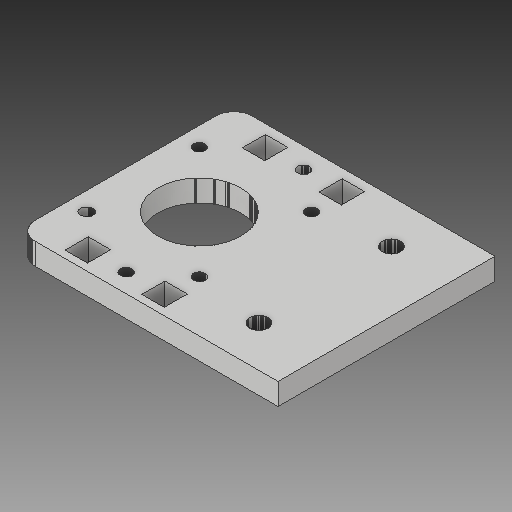
# Autodesk Inventor part: Y-Motor-Mount Top
Saved by Autodesk Inventor 2018 (Build 220112000, 112)
## iProperties
Created: 2016-07-22
Part Number: Y-Motor-Mount Top
Material: Generic
Document SubType Name: Modeling
Designer: User
Density: 1 g/cm^3
Appearance: Default
Mass: 21.9439 g
Surface Area: 104.712 cm^2
Volume: 21.9439 cm^3
Author: User
Autodesk Inventor part; units mm, degrees
ref_plane "YZ Plane" through (0, 0, 0) normal (1, 0, 0) x (0, 1, 0)
ref_plane "XZ Plane" through (0, 0, 0) normal (0, 1, 0) x (-1, 0, 0)
ref_plane "XY Plane" through (0, 0, 0) normal (0, 0, 1) x (1, 0, 0)
sketch "Sketch1" plane through (0, 0, 0) normal (0, 1, 0) x (-1, 0, 0)
  line L0 (968.8679, 195.3235) -> (968.6178, 195.9235)
  line L1 (968.6178, 195.9235) -> (968.2179, 196.4485)
  line L2 (968.2179, 196.4485) -> (967.6929, 196.8485)
  line L3 (967.6929, 196.8485) -> (967.0929, 197.0985)
  line L4 (967.0929, 197.0985) -> (966.4429, 197.1985)
  line L5 (966.4429, 197.1985) -> (965.7929, 197.0984)
  line L6 (965.7929, 197.0984) -> (965.1679, 196.8484)
  line L7 (965.1679, 196.8484) -> (964.6429, 196.4484)
  line L8 (964.6429, 196.4484) -> (964.2429, 195.9234)
  line L9 (964.2429, 195.9234) -> (963.9929, 195.3234)
  line L10 (963.9929, 195.3234) -> (963.9179, 194.6734)
  line L11 (963.9179, 194.6734) -> (963.9929, 194.0234)
  line L12 (963.9929, 194.0234) -> (964.243, 193.3984)
  line L13 (964.243, 193.3984) -> (964.6429, 192.8984)
  line L14 (964.6429, 192.8984) -> (965.1679, 192.4985)
  line L15 (965.1679, 192.4985) -> (965.793, 192.2485)
  line L16 (965.793, 192.2485) -> (966.443, 192.1486)
  line L17 (966.443, 192.1486) -> (967.093, 192.2486)
  line L18 (967.093, 192.2486) -> (967.6929, 192.4987)
  line L19 (967.6929, 192.4987) -> (968.218, 192.8987)
  line L20 (968.218, 192.8987) -> (968.6181, 193.3986)
  line L21 (968.6181, 193.3986) -> (968.868, 194.0236)
  line L22 (968.868, 194.0236) -> (968.9429, 194.6733)
  line L23 (968.9429, 194.6733) -> (968.8679, 195.3235)
  line L24 (983.267, 191.6734) -> (983.267, 185.2734)
  line L25 (983.267, 185.2734) -> (989.467, 185.2734)
  line L26 (989.467, 185.2734) -> (989.467, 191.6734)
  line L27 (989.467, 191.6734) -> (983.267, 191.6734)
  line L28 (987.3418, 197.698) -> (987.3418, 197.798)
  line L29 (987.3418, 197.798) -> (987.3169, 197.898)
  line L30 (987.3169, 197.898) -> (987.2669, 197.998)
  line L31 (987.2669, 197.998) -> (987.2419, 198.098)
  line L32 (987.2419, 198.098) -> (987.1919, 198.198)
  line L33 (987.1919, 198.198) -> (987.1419, 198.298)
  line L34 (987.1419, 198.298) -> (987.0919, 198.373)
  line L35 (987.0919, 198.373) -> (987.042, 198.473)
  line L36 (987.042, 198.473) -> (986.9669, 198.548)
  line L37 (986.9669, 198.548) -> (986.892, 198.6231)
  line L38 (986.892, 198.6231) -> (986.817, 198.6981)
  line L39 (986.817, 198.6981) -> (986.742, 198.7481)
  line L40 (986.742, 198.7481) -> (986.642, 198.8231)
  line L41 (986.642, 198.8231) -> (986.567, 198.8731)
  line L42 (986.567, 198.8731) -> (986.467, 198.9232)
  line L43 (986.467, 198.9232) -> (986.3671, 198.9732)
  line L44 (986.3671, 198.9732) -> (986.2671, 198.9983)
  line L45 (986.2671, 198.9983) -> (986.1671, 199.0483)
  line L46 (986.1671, 199.0483) -> (986.0671, 199.0483)
  line L47 (986.0671, 199.0483) -> (985.9671, 199.0734)
  line L48 (985.9671, 199.0734) -> (985.8671, 199.0983)
  line L49 (985.8671, 199.0983) -> (985.7671, 199.0983)
  line L50 (985.7671, 199.0983) -> (985.6671, 199.0983)
  line L51 (985.6671, 199.0983) -> (985.5422, 199.0734)
  line L52 (985.5422, 199.0734) -> (985.4421, 199.0483)
  line L53 (985.4421, 199.0483) -> (985.3421, 199.0483)
  line L54 (985.3421, 199.0483) -> (985.2421, 198.9983)
  line L55 (985.2421, 198.9983) -> (985.1421, 198.9733)
  line L56 (985.1421, 198.9733) -> (985.0421, 198.9234)
  line L57 (985.0421, 198.9234) -> (984.9671, 198.8733)
  line L58 (984.9671, 198.8733) -> (984.8671, 198.8234)
  line L59 (984.8671, 198.8234) -> (984.7922, 198.7484)
  line L60 (984.7922, 198.7484) -> (984.7171, 198.6984)
  line L61 (984.7171, 198.6984) -> (984.6421, 198.6234)
  line L62 (984.6421, 198.6234) -> (984.5671, 198.5484)
  line L63 (984.5671, 198.5484) -> (984.4921, 198.4734)
  line L64 (984.4921, 198.4734) -> (984.4421, 198.3734)
  line L65 (984.4421, 198.3734) -> (984.3671, 198.2984)
  line L66 (984.3671, 198.2984) -> (984.317, 198.1984)
  line L67 (984.317, 198.1984) -> (984.292, 198.0984)
  line L68 (984.292, 198.0984) -> (984.2421, 197.9984)
  line L69 (984.2421, 197.9984) -> (984.2171, 197.8985)
  line L70 (984.2171, 197.8985) -> (984.192, 197.7984)
  line L71 (984.192, 197.7984) -> (984.167, 197.6984)
  line L72 (984.167, 197.6984) -> (984.167, 197.5984)
  line L73 (984.167, 197.5984) -> (984.167, 197.4984)
  line L74 (984.167, 197.4984) -> (984.167, 197.3984)
  line L75 (984.167, 197.3984) -> (984.167, 197.2734)
  line L76 (984.167, 197.2734) -> (984.192, 197.1734)
  line L77 (984.192, 197.1734) -> (984.2171, 197.0734)
  line L78 (984.2171, 197.0734) -> (984.2421, 196.9734)
  line L79 (984.2421, 196.9734) -> (984.2921, 196.8734)
  line L80 (984.2921, 196.8734) -> (984.317, 196.7734)
  line L81 (984.317, 196.7734) -> (984.3671, 196.6985)
  line L82 (984.3671, 196.6985) -> (984.4421, 196.5985)
  line L83 (984.4421, 196.5985) -> (984.4921, 196.5235)
  line L84 (984.4921, 196.5235) -> (984.5671, 196.4235)
  line L85 (984.5671, 196.4235) -> (984.6421, 196.3485)
  line L86 (984.6421, 196.3485) -> (984.7171, 196.2984)
  line L87 (984.7171, 196.2984) -> (984.7921, 196.2234)
  line L88 (984.7921, 196.2234) -> (984.867, 196.1484)
  line L89 (984.867, 196.1484) -> (984.967, 196.0983)
  line L90 (984.967, 196.0983) -> (985.042, 196.0483)
  line L91 (985.042, 196.0483) -> (985.142, 196.0233)
  line L92 (985.142, 196.0233) -> (985.2419, 195.9732)
  line L93 (985.2419, 195.9732) -> (985.3419, 195.9482)
  line L94 (985.3419, 195.9482) -> (985.4419, 195.9231)
  line L95 (985.4419, 195.9231) -> (985.542, 195.8981)
  line L96 (985.542, 195.8981) -> (985.6669, 195.8981)
  line L97 (985.6669, 195.8981) -> (985.7669, 195.8981)
  line L98 (985.7669, 195.8981) -> (985.8669, 195.8981)
  line L99 (985.8669, 195.8981) -> (985.9669, 195.8981)
  line L100 (985.9669, 195.8981) -> (986.0669, 195.9231)
  line L101 (986.0669, 195.9231) -> (986.1669, 195.9481)
  line L102 (986.1669, 195.9481) -> (986.2669, 195.9731)
  line L103 (986.2669, 195.9731) -> (986.3669, 196.0231)
  line L104 (986.3669, 196.0231) -> (986.4669, 196.0482)
  line L105 (986.4669, 196.0482) -> (986.5669, 196.0981)
  line L106 (986.5669, 196.0981) -> (986.6419, 196.1481)
  line L107 (986.6419, 196.1481) -> (986.7419, 196.2231)
  line L108 (986.7419, 196.2231) -> (986.8169, 196.2981)
  line L109 (986.8169, 196.2981) -> (986.8919, 196.3481)
  line L110 (986.8919, 196.3481) -> (986.9669, 196.4231)
  line L111 (986.9669, 196.4231) -> (987.042, 196.5231)
  line L112 (987.042, 196.5231) -> (987.092, 196.5981)
  line L113 (987.092, 196.5981) -> (987.1419, 196.6981)
  line L114 (987.1419, 196.6981) -> (987.192, 196.7731)
  line L115 (987.192, 196.7731) -> (987.242, 196.8731)
  line L116 (987.242, 196.8731) -> (987.267, 196.9731)
  line L117 (987.267, 196.9731) -> (987.3169, 197.0731)
  line L118 (987.3169, 197.0731) -> (987.3419, 197.1731)
  line L119 (987.3419, 197.1731) -> (987.3419, 197.2731)
  line L120 (987.3419, 197.2731) -> (987.3669, 197.398)
  line L121 (987.3669, 197.398) -> (987.3669, 197.4979)
  line L122 (987.3669, 197.4979) -> (987.3669, 197.598)
  line L123 (987.3669, 197.598) -> (987.3418, 197.698)
  line L124 (1012.7431, 213.7485) -> (1012.6681, 214.4985)
  line L125 (1012.6681, 214.4985) -> (1012.5425, 215.2239)
  line L126 (1012.5425, 215.2239) -> (1012.3674, 215.9738)
  line L127 (1012.3674, 215.9738) -> (1012.1423, 216.6988)
  line L128 (1012.1423, 216.6988) -> (1011.8923, 217.3988)
  line L129 (1011.8923, 217.3988) -> (1011.5673, 218.0738)
  line L130 (1011.5673, 218.0738) -> (1011.2173, 218.7488)
  line L131 (1011.2173, 218.7488) -> (1010.8173, 219.3738)
  line L132 (1010.8173, 219.3738) -> (1010.3922, 219.9987)
  line L133 (1010.3922, 219.9987) -> (1009.917, 220.5735)
  line L134 (1009.917, 220.5735) -> (1009.3919, 221.1234)
  line L135 (1009.3919, 221.1234) -> (1008.8419, 221.6485)
  line L136 (1008.8419, 221.6485) -> (1008.2669, 222.1234)
  line L137 (1008.2669, 222.1234) -> (1007.6419, 222.5484)
  line L138 (1007.6419, 222.5484) -> (1007.0169, 222.9484)
  line L139 (1007.0169, 222.9484) -> (1006.3419, 223.2984)
  line L140 (1006.3419, 223.2984) -> (1005.6669, 223.6234)
  line L141 (1005.6669, 223.6234) -> (1004.967, 223.8735)
  line L142 (1004.967, 223.8735) -> (1004.2419, 224.0985)
  line L143 (1004.2419, 224.0985) -> (1003.5169, 224.2736)
  line L144 (1003.5169, 224.2736) -> (1002.7669, 224.3986)
  line L145 (1002.7669, 224.3986) -> (1002.017, 224.4737)
  line L146 (1002.017, 224.4737) -> (1001.267, 224.4987)
  line L147 (1001.267, 224.4987) -> (1000.517, 224.4737)
  line L148 (1000.517, 224.4737) -> (999.767, 224.3986)
  line L149 (999.767, 224.3986) -> (999.017, 224.2737)
  line L150 (999.017, 224.2737) -> (998.2919, 224.0987)
  line L151 (998.2919, 224.0987) -> (997.5669, 223.8736)
  line L152 (997.5669, 223.8736) -> (996.8669, 223.6236)
  line L153 (996.8669, 223.6236) -> (996.1669, 223.2986)
  line L154 (996.1669, 223.2986) -> (995.5169, 222.9486)
  line L155 (995.5169, 222.9486) -> (994.8669, 222.5486)
  line L156 (994.8669, 222.5486) -> (994.2671, 222.1234)
  line L157 (994.2671, 222.1234) -> (993.6672, 221.6483)
  line L158 (993.6672, 221.6483) -> (993.142, 221.1234)
  line L159 (993.142, 221.1234) -> (992.617, 220.5734)
  line L160 (992.617, 220.5734) -> (992.142, 219.9984)
  line L161 (992.142, 219.9984) -> (991.692, 219.3735)
  line L162 (991.692, 219.3735) -> (991.292, 218.7484)
  line L163 (991.292, 218.7484) -> (990.942, 218.0734)
  line L164 (990.942, 218.0734) -> (990.642, 217.3984)
  line L165 (990.642, 217.3984) -> (990.367, 216.6984)
  line L166 (990.367, 216.6984) -> (990.142, 215.9734)
  line L167 (990.142, 215.9734) -> (989.992, 215.2234)
  line L168 (989.992, 215.2234) -> (989.8671, 214.4984)
  line L169 (989.8671, 214.4984) -> (989.792, 213.7484)
  line L170 (989.792, 213.7484) -> (989.767, 212.9984)
  line L171 (989.767, 212.9984) -> (989.792, 212.2484)
  line L172 (989.792, 212.2484) -> (989.8671, 211.4984)
  line L173 (989.8671, 211.4984) -> (989.992, 210.7484)
  line L174 (989.992, 210.7484) -> (990.142, 210.0234)
  line L175 (990.142, 210.0234) -> (990.367, 209.2984)
  line L176 (990.367, 209.2984) -> (990.642, 208.5984)
  line L177 (990.642, 208.5984) -> (990.942, 207.8984)
  line L178 (990.942, 207.8984) -> (991.292, 207.2484)
  line L179 (991.292, 207.2484) -> (991.692, 206.5984)
  line L180 (991.692, 206.5984) -> (992.1421, 205.9985)
  line L181 (992.1421, 205.9985) -> (992.6172, 205.3986)
  line L182 (992.6172, 205.3986) -> (993.1424, 204.8487)
  line L183 (993.1424, 204.8487) -> (993.6674, 204.3488)
  line L184 (993.6674, 204.3488) -> (994.2675, 203.8739)
  line L185 (994.2675, 203.8739) -> (994.8673, 203.4237)
  line L186 (994.8673, 203.4237) -> (995.5172, 203.0235)
  line L187 (995.5172, 203.0235) -> (996.1671, 202.6732)
  line L188 (996.1671, 202.6732) -> (996.8669, 202.373)
  line L189 (996.8669, 202.373) -> (997.567, 202.098)
  line L190 (997.567, 202.098) -> (998.292, 201.8729)
  line L191 (998.292, 201.8729) -> (999.017, 201.7229)
  line L192 (999.017, 201.7229) -> (999.767, 201.5978)
  line L193 (999.767, 201.5978) -> (1000.517, 201.5228)
  line L194 (1000.517, 201.5228) -> (1001.267, 201.4978)
  line L195 (1001.267, 201.4978) -> (1002.017, 201.5228)
  line L196 (1002.017, 201.5228) -> (1002.767, 201.5978)
  line L197 (1002.767, 201.5978) -> (1003.517, 201.7228)
  line L198 (1003.517, 201.7228) -> (1004.242, 201.8727)
  line L199 (1004.242, 201.8727) -> (1004.967, 202.0978)
  line L200 (1004.967, 202.0978) -> (1005.6669, 202.3728)
  line L201 (1005.6669, 202.3728) -> (1006.3419, 202.6728)
  line L202 (1006.3419, 202.6728) -> (1007.017, 203.0228)
  line L203 (1007.017, 203.0228) -> (1007.6419, 203.4228)
  line L204 (1007.6419, 203.4228) -> (1008.2669, 203.8728)
  line L205 (1008.2669, 203.8728) -> (1008.8419, 204.3478)
  line L206 (1008.8419, 204.3478) -> (1009.3919, 204.8478)
  line L207 (1009.3919, 204.8478) -> (1009.9169, 205.3978)
  line L208 (1009.9169, 205.3978) -> (1010.3921, 205.9977)
  line L209 (1010.3921, 205.9977) -> (1010.8171, 206.5977)
  line L210 (1010.8171, 206.5977) -> (1011.2173, 207.2475)
  line L211 (1011.2173, 207.2475) -> (1011.5675, 207.8974)
  line L212 (1011.5675, 207.8974) -> (1011.8928, 208.5973)
  line L213 (1011.8928, 208.5973) -> (1012.1428, 209.2973)
  line L214 (1012.1428, 209.2973) -> (1012.3679, 210.0223)
  line L215 (1012.3679, 210.0223) -> (1012.5429, 210.7473)
  line L216 (1012.5429, 210.7473) -> (1012.6679, 211.4973)
  line L217 (1012.6679, 211.4973) -> (1012.743, 212.2473)
  line L218 (1012.743, 212.2473) -> (1012.7681, 212.9999)
  line L219 (1012.7681, 212.9999) -> (1012.7431, 213.7485)
  line L220 (998.542, 188.6729) -> (998.542, 188.7729)
  line L221 (998.542, 188.7729) -> (998.5169, 188.8729)
  line L222 (998.5169, 188.8729) -> (998.467, 188.9729)
  line L223 (998.467, 188.9729) -> (998.442, 189.0729)
  line L224 (998.442, 189.0729) -> (998.392, 189.1729)
  line L225 (998.392, 189.1729) -> (998.342, 189.2729)
  line L226 (998.342, 189.2729) -> (998.292, 189.3479)
  line L227 (998.292, 189.3479) -> (998.242, 189.4479)
  line L228 (998.242, 189.4479) -> (998.167, 189.523)
  line L229 (998.167, 189.523) -> (998.092, 189.598)
  line L230 (998.092, 189.598) -> (998.0171, 189.673)
  line L231 (998.0171, 189.673) -> (997.9421, 189.748)
  line L232 (997.9421, 189.748) -> (997.8421, 189.7981)
  line L233 (997.8421, 189.7981) -> (997.7671, 189.8481)
  line L234 (997.7671, 189.8481) -> (997.6671, 189.8982)
  line L235 (997.6671, 189.8982) -> (997.5671, 189.9482)
  line L236 (997.5671, 189.9482) -> (997.4672, 189.9732)
  line L237 (997.4672, 189.9732) -> (997.3672, 190.0233)
  line L238 (997.3672, 190.0233) -> (997.2672, 190.0483)
  line L239 (997.2672, 190.0483) -> (997.1672, 190.0483)
  line L240 (997.1672, 190.0483) -> (997.0672, 190.0734)
  line L241 (997.0672, 190.0734) -> (996.9672, 190.0734)
  line L242 (996.9672, 190.0734) -> (996.8671, 190.0734)
  line L243 (996.8671, 190.0734) -> (996.7422, 190.0483)
  line L244 (996.7422, 190.0483) -> (996.6421, 190.0483)
  line L245 (996.6421, 190.0483) -> (996.5422, 190.0233)
  line L246 (996.5422, 190.0233) -> (996.4421, 189.9733)
  line L247 (996.4421, 189.9733) -> (996.3421, 189.9483)
  line L248 (996.3421, 189.9483) -> (996.2421, 189.8984)
  line L249 (996.2421, 189.8984) -> (996.1671, 189.8484)
  line L250 (996.1671, 189.8484) -> (996.0671, 189.7984)
  line L251 (996.0671, 189.7984) -> (995.9921, 189.7484)
  line L252 (995.9921, 189.7484) -> (995.9171, 189.6734)
  line L253 (995.9171, 189.6734) -> (995.8421, 189.5984)
  line L254 (995.8421, 189.5984) -> (995.7671, 189.5234)
  line L255 (995.7671, 189.5234) -> (995.6921, 189.4484)
  line L256 (995.6921, 189.4484) -> (995.6421, 189.3484)
  line L257 (995.6421, 189.3484) -> (995.5671, 189.2734)
  line L258 (995.5671, 189.2734) -> (995.5171, 189.1734)
  line L259 (995.5171, 189.1734) -> (995.4921, 189.0734)
  line L260 (995.4921, 189.0734) -> (995.4421, 188.9734)
  line L261 (995.4421, 188.9734) -> (995.417, 188.8734)
  line L262 (995.417, 188.8734) -> (995.3921, 188.7734)
  line L263 (995.3921, 188.7734) -> (995.3671, 188.6734)
  line L264 (995.3671, 188.6734) -> (995.3671, 188.5734)
  line L265 (995.3671, 188.5734) -> (995.3671, 188.4734)
  line L266 (995.3671, 188.4734) -> (995.3671, 188.3735)
  line L267 (995.3671, 188.3735) -> (995.3671, 188.2734)
  line L268 (995.3671, 188.2734) -> (995.392, 188.1484)
  line L269 (995.392, 188.1484) -> (995.417, 188.0484)
  line L270 (995.417, 188.0484) -> (995.4421, 187.9484)
  line L271 (995.4421, 187.9484) -> (995.4921, 187.8484)
  line L272 (995.4921, 187.8484) -> (995.517, 187.7735)
  line L273 (995.517, 187.7735) -> (995.5671, 187.6734)
  line L274 (995.5671, 187.6734) -> (995.6421, 187.5734)
  line L275 (995.6421, 187.5734) -> (995.6921, 187.4984)
  line L276 (995.6921, 187.4984) -> (995.767, 187.4234)
  line L277 (995.767, 187.4234) -> (995.842, 187.3484)
  line L278 (995.842, 187.3484) -> (995.9169, 187.2733)
  line L279 (995.9169, 187.2733) -> (995.9919, 187.1983)
  line L280 (995.9919, 187.1983) -> (996.0669, 187.1483)
  line L281 (996.0669, 187.1483) -> (996.1669, 187.0733)
  line L282 (996.1669, 187.0733) -> (996.2419, 187.0233)
  line L283 (996.2419, 187.0233) -> (996.3419, 186.9982)
  line L284 (996.3419, 186.9982) -> (996.4418, 186.9482)
  line L285 (996.4418, 186.9482) -> (996.5419, 186.9232)
  line L286 (996.5419, 186.9232) -> (996.6418, 186.8981)
  line L287 (996.6418, 186.8981) -> (996.7419, 186.8731)
  line L288 (996.7419, 186.8731) -> (996.8668, 186.8731)
  line L289 (996.8668, 186.8731) -> (996.9669, 186.8731)
  line L290 (996.9669, 186.8731) -> (997.0669, 186.8731)
  line L291 (997.0669, 186.8731) -> (997.1668, 186.8731)
  line L292 (997.1668, 186.8731) -> (997.2668, 186.8981)
  line L293 (997.2668, 186.8981) -> (997.3668, 186.9231)
  line L294 (997.3668, 186.9231) -> (997.4668, 186.9481)
  line L295 (997.4668, 186.9481) -> (997.5668, 186.9981)
  line L296 (997.5668, 186.9981) -> (997.6668, 187.0231)
  line L297 (997.6668, 187.0231) -> (997.7668, 187.0731)
  line L298 (997.7668, 187.0731) -> (997.8418, 187.1481)
  line L299 (997.8418, 187.1481) -> (997.9418, 187.198)
  line L300 (997.9418, 187.198) -> (998.0169, 187.273)
  line L301 (998.0169, 187.273) -> (998.0919, 187.348)
  line L302 (998.0919, 187.348) -> (998.1669, 187.423)
  line L303 (998.1669, 187.423) -> (998.242, 187.498)
  line L304 (998.242, 187.498) -> (998.2919, 187.573)
  line L305 (998.2919, 187.573) -> (998.3419, 187.673)
  line L306 (998.3419, 187.673) -> (998.392, 187.773)
  line L307 (998.392, 187.773) -> (998.442, 187.848)
  line L308 (998.442, 187.848) -> (998.467, 187.948)
  line L309 (998.467, 187.948) -> (998.5169, 188.048)
  line L310 (998.5169, 188.048) -> (998.542, 188.148)
  line L311 (998.542, 188.148) -> (998.542, 188.273)
  line L312 (998.542, 188.273) -> (998.567, 188.373)
  line L313 (998.567, 188.373) -> (998.567, 188.473)
  line L314 (998.567, 188.473) -> (998.567, 188.5729)
  line L315 (998.567, 188.5729) -> (998.542, 188.6729)
  line L316 (1004.467, 191.6734) -> (1004.467, 185.2734)
  line L317 (1004.467, 185.2734) -> (1010.667, 185.2734)
  line L318 (1010.667, 185.2734) -> (1010.667, 191.6734)
  line L319 (1010.667, 191.6734) -> (1004.467, 191.6734)
  line L320 (1018.3418, 197.698) -> (1018.3418, 197.798)
  line L321 (1018.3418, 197.798) -> (1018.3168, 197.8981)
  line L322 (1018.3168, 197.8981) -> (1018.2669, 197.998)
  line L323 (1018.2669, 197.998) -> (1018.2419, 198.098)
  line L324 (1018.2419, 198.098) -> (1018.1919, 198.198)
  line L325 (1018.1919, 198.198) -> (1018.1418, 198.2981)
  line L326 (1018.1418, 198.2981) -> (1018.0919, 198.373)
  line L327 (1018.0919, 198.373) -> (1018.0419, 198.4731)
  line L328 (1018.0419, 198.4731) -> (1017.9669, 198.5481)
  line L329 (1017.9669, 198.5481) -> (1017.892, 198.6231)
  line L330 (1017.892, 198.6231) -> (1017.817, 198.6981)
  line L331 (1017.817, 198.6981) -> (1017.742, 198.7482)
  line L332 (1017.742, 198.7482) -> (1017.642, 198.8232)
  line L333 (1017.642, 198.8232) -> (1017.567, 198.8732)
  line L334 (1017.567, 198.8732) -> (1017.467, 198.9233)
  line L335 (1017.467, 198.9233) -> (1017.367, 198.9733)
  line L336 (1017.367, 198.9733) -> (1017.2671, 198.9983)
  line L337 (1017.2671, 198.9983) -> (1017.1671, 199.0484)
  line L338 (1017.1671, 199.0484) -> (1017.0671, 199.0484)
  line L339 (1017.0671, 199.0484) -> (1016.9671, 199.0734)
  line L340 (1016.9671, 199.0734) -> (1016.8671, 199.0984)
  line L341 (1016.8671, 199.0984) -> (1016.7671, 199.0984)
  line L342 (1016.7671, 199.0984) -> (1016.6671, 199.0984)
  line L343 (1016.6671, 199.0984) -> (1016.5422, 199.0734)
  line L344 (1016.5422, 199.0734) -> (1016.4421, 199.0484)
  line L345 (1016.4421, 199.0484) -> (1016.3421, 199.0484)
  line L346 (1016.3421, 199.0484) -> (1016.2421, 198.9984)
  line L347 (1016.2421, 198.9984) -> (1016.1421, 198.9734)
  line L348 (1016.1421, 198.9734) -> (1016.0421, 198.9234)
  line L349 (1016.0421, 198.9234) -> (1015.9672, 198.8734)
  line L350 (1015.9672, 198.8734) -> (1015.8671, 198.8234)
  line L351 (1015.8671, 198.8234) -> (1015.7922, 198.7484)
  line L352 (1015.7922, 198.7484) -> (1015.7171, 198.6984)
  line L353 (1015.7171, 198.6984) -> (1015.6422, 198.6234)
  line L354 (1015.6422, 198.6234) -> (1015.5671, 198.5484)
  line L355 (1015.5671, 198.5484) -> (1015.4921, 198.4734)
  line L356 (1015.4921, 198.4734) -> (1015.4421, 198.3734)
  line L357 (1015.4421, 198.3734) -> (1015.3671, 198.2984)
  line L358 (1015.3671, 198.2984) -> (1015.317, 198.1984)
  line L359 (1015.317, 198.1984) -> (1015.2921, 198.0984)
  line L360 (1015.2921, 198.0984) -> (1015.242, 197.9984)
  line L361 (1015.242, 197.9984) -> (1015.217, 197.8984)
  line L362 (1015.217, 197.8984) -> (1015.192, 197.7984)
  line L363 (1015.192, 197.7984) -> (1015.167, 197.6984)
  line L364 (1015.167, 197.6984) -> (1015.167, 197.5984)
  line L365 (1015.167, 197.5984) -> (1015.167, 197.4984)
  line L366 (1015.167, 197.4984) -> (1015.167, 197.3984)
  line L367 (1015.167, 197.3984) -> (1015.167, 197.2734)
  line L368 (1015.167, 197.2734) -> (1015.192, 197.1734)
  line L369 (1015.192, 197.1734) -> (1015.217, 197.0734)
  line L370 (1015.217, 197.0734) -> (1015.242, 196.9734)
  line L371 (1015.242, 196.9734) -> (1015.292, 196.8734)
  line L372 (1015.292, 196.8734) -> (1015.317, 196.7734)
  line L373 (1015.317, 196.7734) -> (1015.3671, 196.6984)
  line L374 (1015.3671, 196.6984) -> (1015.4421, 196.5984)
  line L375 (1015.4421, 196.5984) -> (1015.4921, 196.5234)
  line L376 (1015.4921, 196.5234) -> (1015.5671, 196.4235)
  line L377 (1015.5671, 196.4235) -> (1015.6421, 196.3485)
  line L378 (1015.6421, 196.3485) -> (1015.717, 196.2984)
  line L379 (1015.717, 196.2984) -> (1015.7921, 196.2234)
  line L380 (1015.7921, 196.2234) -> (1015.867, 196.1484)
  line L381 (1015.867, 196.1484) -> (1015.9671, 196.0984)
  line L382 (1015.9671, 196.0984) -> (1016.042, 196.0484)
  line L383 (1016.042, 196.0484) -> (1016.142, 196.0233)
  line L384 (1016.142, 196.0233) -> (1016.2419, 195.9733)
  line L385 (1016.2419, 195.9733) -> (1016.3419, 195.9482)
  line L386 (1016.3419, 195.9482) -> (1016.4419, 195.9232)
  line L387 (1016.4419, 195.9232) -> (1016.542, 195.8982)
  line L388 (1016.542, 195.8982) -> (1016.667, 195.8982)
  line L389 (1016.667, 195.8982) -> (1016.7669, 195.8982)
  line L390 (1016.7669, 195.8982) -> (1016.8669, 195.8982)
  line L391 (1016.8669, 195.8982) -> (1016.9669, 195.8982)
  line L392 (1016.9669, 195.8982) -> (1017.0669, 195.9231)
  line L393 (1017.0669, 195.9231) -> (1017.1669, 195.9482)
  line L394 (1017.1669, 195.9482) -> (1017.2669, 195.9732)
  line L395 (1017.2669, 195.9732) -> (1017.3669, 196.0232)
  line L396 (1017.3669, 196.0232) -> (1017.4669, 196.0482)
  line L397 (1017.4669, 196.0482) -> (1017.5669, 196.0982)
  line L398 (1017.5669, 196.0982) -> (1017.6419, 196.1481)
  line L399 (1017.6419, 196.1481) -> (1017.7419, 196.2232)
  line L400 (1017.7419, 196.2232) -> (1017.8169, 196.2981)
  line L401 (1017.8169, 196.2981) -> (1017.892, 196.3482)
  line L402 (1017.892, 196.3482) -> (1017.9669, 196.4232)
  line L403 (1017.9669, 196.4232) -> (1018.0419, 196.5231)
  line L404 (1018.0419, 196.5231) -> (1018.0919, 196.5981)
  line L405 (1018.0919, 196.5981) -> (1018.1419, 196.6982)
  line L406 (1018.1419, 196.6982) -> (1018.1919, 196.7731)
  line L407 (1018.1919, 196.7731) -> (1018.242, 196.8731)
  line L408 (1018.242, 196.8731) -> (1018.267, 196.9731)
  line L409 (1018.267, 196.9731) -> (1018.3169, 197.0731)
  line L410 (1018.3169, 197.0731) -> (1018.3419, 197.1731)
  line L411 (1018.3419, 197.1731) -> (1018.3419, 197.2731)
  line L412 (1018.3419, 197.2731) -> (1018.3669, 197.3981)
  line L413 (1018.3669, 197.3981) -> (1018.3669, 197.498)
  line L414 (1018.3669, 197.498) -> (1018.3669, 197.5981)
  line L415 (1018.3669, 197.5981) -> (1018.3418, 197.698)
  line L416 (1018.3419, 228.698) -> (1018.3419, 228.798)
  line L417 (1018.3419, 228.798) -> (1018.3169, 228.898)
  line L418 (1018.3169, 228.898) -> (1018.2669, 228.998)
  line L419 (1018.2669, 228.998) -> (1018.2419, 229.098)
  line L420 (1018.2419, 229.098) -> (1018.1919, 229.198)
  line L421 (1018.1919, 229.198) -> (1018.1419, 229.298)
  line L422 (1018.1419, 229.298) -> (1018.0919, 229.373)
  line L423 (1018.0919, 229.373) -> (1018.0419, 229.473)
  line L424 (1018.0419, 229.473) -> (1017.9669, 229.548)
  line L425 (1017.9669, 229.548) -> (1017.892, 229.623)
  line L426 (1017.892, 229.623) -> (1017.817, 229.6981)
  line L427 (1017.817, 229.6981) -> (1017.742, 229.7481)
  line L428 (1017.742, 229.7481) -> (1017.6421, 229.8231)
  line L429 (1017.6421, 229.8231) -> (1017.5671, 229.8731)
  line L430 (1017.5671, 229.8731) -> (1017.4671, 229.9232)
  line L431 (1017.4671, 229.9232) -> (1017.3671, 229.9732)
  line L432 (1017.3671, 229.9732) -> (1017.2671, 229.9983)
  line L433 (1017.2671, 229.9983) -> (1017.1671, 230.0483)
  line L434 (1017.1671, 230.0483) -> (1017.0672, 230.0483)
  line L435 (1017.0672, 230.0483) -> (1016.9672, 230.0734)
  line L436 (1016.9672, 230.0734) -> (1016.8672, 230.0983)
  line L437 (1016.8672, 230.0983) -> (1016.7672, 230.0983)
  line L438 (1016.7672, 230.0983) -> (1016.6672, 230.0983)
  line L439 (1016.6672, 230.0983) -> (1016.5422, 230.0734)
  line L440 (1016.5422, 230.0734) -> (1016.4421, 230.0483)
  line L441 (1016.4421, 230.0483) -> (1016.3421, 230.0483)
  line L442 (1016.3421, 230.0483) -> (1016.2421, 229.9984)
  line L443 (1016.2421, 229.9984) -> (1016.1421, 229.9734)
  line L444 (1016.1421, 229.9734) -> (1016.0422, 229.9234)
  line L445 (1016.0422, 229.9234) -> (1015.9672, 229.8733)
  line L446 (1015.9672, 229.8733) -> (1015.8671, 229.8233)
  line L447 (1015.8671, 229.8233) -> (1015.7922, 229.7483)
  line L448 (1015.7922, 229.7483) -> (1015.7171, 229.6984)
  line L449 (1015.7171, 229.6984) -> (1015.6421, 229.6234)
  line L450 (1015.6421, 229.6234) -> (1015.5671, 229.5484)
  line L451 (1015.5671, 229.5484) -> (1015.4921, 229.4734)
  line L452 (1015.4921, 229.4734) -> (1015.4421, 229.3734)
  line L453 (1015.4421, 229.3734) -> (1015.3671, 229.2984)
  line L454 (1015.3671, 229.2984) -> (1015.3171, 229.1984)
  line L455 (1015.3171, 229.1984) -> (1015.2921, 229.0984)
  line L456 (1015.2921, 229.0984) -> (1015.242, 228.9984)
  line L457 (1015.242, 228.9984) -> (1015.217, 228.8985)
  line L458 (1015.217, 228.8985) -> (1015.192, 228.7984)
  line L459 (1015.192, 228.7984) -> (1015.167, 228.6984)
  line L460 (1015.167, 228.6984) -> (1015.167, 228.5984)
  line L461 (1015.167, 228.5984) -> (1015.167, 228.4984)
  line L462 (1015.167, 228.4984) -> (1015.167, 228.3984)
  line L463 (1015.167, 228.3984) -> (1015.167, 228.2734)
  line L464 (1015.167, 228.2734) -> (1015.192, 228.1735)
  line L465 (1015.192, 228.1735) -> (1015.217, 228.0734)
  line L466 (1015.217, 228.0734) -> (1015.242, 227.9734)
  line L467 (1015.242, 227.9734) -> (1015.292, 227.8734)
  line L468 (1015.292, 227.8734) -> (1015.317, 227.7734)
  line L469 (1015.317, 227.7734) -> (1015.3671, 227.6984)
  line L470 (1015.3671, 227.6984) -> (1015.4421, 227.5984)
  line L471 (1015.4421, 227.5984) -> (1015.4921, 227.5235)
  line L472 (1015.4921, 227.5235) -> (1015.5671, 227.4235)
  line L473 (1015.5671, 227.4235) -> (1015.6421, 227.3484)
  line L474 (1015.6421, 227.3484) -> (1015.717, 227.2984)
  line L475 (1015.717, 227.2984) -> (1015.7921, 227.2234)
  line L476 (1015.7921, 227.2234) -> (1015.867, 227.1483)
  line L477 (1015.867, 227.1483) -> (1015.9671, 227.0984)
  line L478 (1015.9671, 227.0984) -> (1016.042, 227.0484)
  line L479 (1016.042, 227.0484) -> (1016.142, 227.0233)
  line L480 (1016.142, 227.0233) -> (1016.242, 226.9733)
  line L481 (1016.242, 226.9733) -> (1016.3419, 226.9482)
  line L482 (1016.3419, 226.9482) -> (1016.4419, 226.9232)
  line L483 (1016.4419, 226.9232) -> (1016.542, 226.8982)
  line L484 (1016.542, 226.8982) -> (1016.667, 226.8982)
  line L485 (1016.667, 226.8982) -> (1016.767, 226.8982)
  line L486 (1016.767, 226.8982) -> (1016.867, 226.8982)
  line L487 (1016.867, 226.8982) -> (1016.9669, 226.8982)
  line L488 (1016.9669, 226.8982) -> (1017.0669, 226.9232)
  line L489 (1017.0669, 226.9232) -> (1017.1669, 226.9482)
  line L490 (1017.1669, 226.9482) -> (1017.2669, 226.9732)
  line L491 (1017.2669, 226.9732) -> (1017.3669, 227.0232)
  line L492 (1017.3669, 227.0232) -> (1017.4669, 227.0482)
  line L493 (1017.4669, 227.0482) -> (1017.5669, 227.0982)
  line L494 (1017.5669, 227.0982) -> (1017.6419, 227.1482)
  line L495 (1017.6419, 227.1482) -> (1017.7419, 227.2232)
  line L496 (1017.7419, 227.2232) -> (1017.8169, 227.2982)
  line L497 (1017.8169, 227.2982) -> (1017.8919, 227.3482)
  line L498 (1017.8919, 227.3482) -> (1017.9669, 227.4232)
  line L499 (1017.9669, 227.4232) -> (1018.0419, 227.5232)
  line L500 (1018.0419, 227.5232) -> (1018.092, 227.5982)
  line L501 (1018.092, 227.5982) -> (1018.1419, 227.6982)
  line L502 (1018.1419, 227.6982) -> (1018.1919, 227.7732)
  line L503 (1018.1919, 227.7732) -> (1018.242, 227.8732)
  line L504 (1018.242, 227.8732) -> (1018.267, 227.9731)
  line L505 (1018.267, 227.9731) -> (1018.3169, 228.0732)
  line L506 (1018.3169, 228.0732) -> (1018.3419, 228.1732)
  line L507 (1018.3419, 228.1732) -> (1018.3419, 228.2731)
  line L508 (1018.3419, 228.2731) -> (1018.3669, 228.3982)
  line L509 (1018.3669, 228.3982) -> (1018.3669, 228.4982)
  line L510 (1018.3669, 228.4982) -> (1018.3669, 228.598)
  line L511 (1018.3669, 228.598) -> (1018.3419, 228.698)
  line L512 (1004.467, 240.6984) -> (1004.467, 234.2984)
  line L513 (1004.467, 234.2984) -> (1010.667, 234.2984)
  line L514 (1010.667, 234.2984) -> (1010.667, 240.6984)
  line L515 (1010.667, 240.6984) -> (1004.467, 240.6984)
  line L516 (998.5421, 237.723) -> (998.5421, 237.823)
  line L517 (998.5421, 237.823) -> (998.517, 237.923)
  line L518 (998.517, 237.923) -> (998.467, 238.023)
  line L519 (998.467, 238.023) -> (998.4421, 238.123)
  line L520 (998.4421, 238.123) -> (998.392, 238.223)
  line L521 (998.392, 238.223) -> (998.342, 238.298)
  line L522 (998.342, 238.298) -> (998.292, 238.398)
  line L523 (998.292, 238.398) -> (998.2421, 238.473)
  line L524 (998.2421, 238.473) -> (998.167, 238.573)
  line L525 (998.167, 238.573) -> (998.092, 238.648)
  line L526 (998.092, 238.648) -> (998.017, 238.7231)
  line L527 (998.017, 238.7231) -> (997.942, 238.7731)
  line L528 (997.942, 238.7731) -> (997.8421, 238.8481)
  line L529 (997.8421, 238.8481) -> (997.7671, 238.8981)
  line L530 (997.7671, 238.8981) -> (997.6671, 238.9482)
  line L531 (997.6671, 238.9482) -> (997.5671, 238.9982)
  line L532 (997.5671, 238.9982) -> (997.4671, 239.0233)
  line L533 (997.4671, 239.0233) -> (997.3672, 239.0482)
  line L534 (997.3672, 239.0482) -> (997.2672, 239.0733)
  line L535 (997.2672, 239.0733) -> (997.1672, 239.0984)
  line L536 (997.1672, 239.0984) -> (997.0672, 239.0984)
  line L537 (997.0672, 239.0984) -> (996.9672, 239.0984)
  line L538 (996.9672, 239.0984) -> (996.8671, 239.0984)
  line L539 (996.8671, 239.0984) -> (996.7422, 239.0984)
  line L540 (996.7422, 239.0984) -> (996.6422, 239.0733)
  line L541 (996.6422, 239.0733) -> (996.5422, 239.0483)
  line L542 (996.5422, 239.0483) -> (996.4422, 239.0233)
  line L543 (996.4422, 239.0233) -> (996.3422, 238.9983)
  line L544 (996.3422, 238.9983) -> (996.2422, 238.9483)
  line L545 (996.2422, 238.9483) -> (996.1672, 238.8983)
  line L546 (996.1672, 238.8983) -> (996.0672, 238.8483)
  line L547 (996.0672, 238.8483) -> (995.9921, 238.7733)
  line L548 (995.9921, 238.7733) -> (995.9171, 238.7233)
  line L549 (995.9171, 238.7233) -> (995.8422, 238.6484)
  line L550 (995.8422, 238.6484) -> (995.7672, 238.5734)
  line L551 (995.7672, 238.5734) -> (995.6921, 238.4734)
  line L552 (995.6921, 238.4734) -> (995.6421, 238.3984)
  line L553 (995.6421, 238.3984) -> (995.5671, 238.2984)
  line L554 (995.5671, 238.2984) -> (995.517, 238.2234)
  line L555 (995.517, 238.2234) -> (995.492, 238.1234)
  line L556 (995.492, 238.1234) -> (995.4421, 238.0234)
  line L557 (995.4421, 238.0234) -> (995.417, 237.9234)
  line L558 (995.417, 237.9234) -> (995.3921, 237.8234)
  line L559 (995.3921, 237.8234) -> (995.3671, 237.7234)
  line L560 (995.3671, 237.7234) -> (995.3671, 237.6235)
  line L561 (995.3671, 237.6235) -> (995.3671, 237.4984)
  line L562 (995.3671, 237.4984) -> (995.3671, 237.3985)
  line L563 (995.3671, 237.3985) -> (995.3671, 237.2984)
  line L564 (995.3671, 237.2984) -> (995.3921, 237.1984)
  line L565 (995.3921, 237.1984) -> (995.417, 237.0985)
  line L566 (995.417, 237.0985) -> (995.4421, 236.9984)
  line L567 (995.4421, 236.9984) -> (995.4921, 236.8984)
  line L568 (995.4921, 236.8984) -> (995.5171, 236.7985)
  line L569 (995.5171, 236.7985) -> (995.5671, 236.6984)
  line L570 (995.5671, 236.6984) -> (995.6421, 236.6234)
  line L571 (995.6421, 236.6234) -> (995.692, 236.5484)
  line L572 (995.692, 236.5484) -> (995.7671, 236.4484)
  line L573 (995.7671, 236.4484) -> (995.842, 236.3734)
  line L574 (995.842, 236.3734) -> (995.9169, 236.2983)
  line L575 (995.9169, 236.2983) -> (995.9919, 236.2483)
  line L576 (995.9919, 236.2483) -> (996.0669, 236.1733)
  line L577 (996.0669, 236.1733) -> (996.1669, 236.1233)
  line L578 (996.1669, 236.1233) -> (996.2419, 236.0733)
  line L579 (996.2419, 236.0733) -> (996.3419, 236.0232)
  line L580 (996.3419, 236.0232) -> (996.4419, 235.9982)
  line L581 (996.4419, 235.9982) -> (996.542, 235.9732)
  line L582 (996.542, 235.9732) -> (996.6419, 235.9481)
  line L583 (996.6419, 235.9481) -> (996.7419, 235.9231)
  line L584 (996.7419, 235.9231) -> (996.8668, 235.9231)
  line L585 (996.8668, 235.9231) -> (996.9669, 235.8981)
  line L586 (996.9669, 235.8981) -> (997.0669, 235.9231)
  line L587 (997.0669, 235.9231) -> (997.1669, 235.9231)
  line L588 (997.1669, 235.9231) -> (997.2669, 235.9481)
  line L589 (997.2669, 235.9481) -> (997.3668, 235.9731)
  line L590 (997.3668, 235.9731) -> (997.4668, 235.9981)
  line L591 (997.4668, 235.9981) -> (997.5668, 236.0231)
  line L592 (997.5668, 236.0231) -> (997.6668, 236.0731)
  line L593 (997.6668, 236.0731) -> (997.7668, 236.1231)
  line L594 (997.7668, 236.1231) -> (997.8418, 236.1731)
  line L595 (997.8418, 236.1731) -> (997.9418, 236.2481)
  line L596 (997.9418, 236.2481) -> (998.0168, 236.2981)
  line L597 (998.0168, 236.2981) -> (998.0919, 236.3731)
  line L598 (998.0919, 236.3731) -> (998.1669, 236.448)
  line L599 (998.1669, 236.448) -> (998.242, 236.548)
  line L600 (998.242, 236.548) -> (998.2919, 236.623)
  line L601 (998.2919, 236.623) -> (998.3419, 236.698)
  line L602 (998.3419, 236.698) -> (998.392, 236.798)
  line L603 (998.392, 236.798) -> (998.442, 236.898)
  line L604 (998.442, 236.898) -> (998.467, 236.998)
  line L605 (998.467, 236.998) -> (998.517, 237.098)
  line L606 (998.517, 237.098) -> (998.5421, 237.1979)
  line L607 (998.5421, 237.1979) -> (998.5421, 237.298)
  line L608 (998.5421, 237.298) -> (998.5671, 237.398)
  line L609 (998.5671, 237.398) -> (998.5671, 237.4979)
  line L610 (998.5671, 237.4979) -> (998.5671, 237.623)
  line L611 (998.5671, 237.623) -> (998.5421, 237.723)
  line L612 (983.267, 240.6984) -> (983.267, 234.2984)
  line L613 (983.267, 234.2984) -> (989.467, 234.2984)
  line L614 (989.467, 234.2984) -> (989.467, 240.6984)
  line L615 (989.467, 240.6984) -> (983.267, 240.6984)
  line L616 (987.3418, 228.698) -> (987.3418, 228.798)
  line L617 (987.3418, 228.798) -> (987.3168, 228.898)
  line L618 (987.3168, 228.898) -> (987.2669, 228.998)
  line L619 (987.2669, 228.998) -> (987.2419, 229.098)
  line L620 (987.2419, 229.098) -> (987.1919, 229.1981)
  line L621 (987.1919, 229.1981) -> (987.1419, 229.298)
  line L622 (987.1419, 229.298) -> (987.0919, 229.373)
  line L623 (987.0919, 229.373) -> (987.0419, 229.473)
  line L624 (987.0419, 229.473) -> (986.9669, 229.5481)
  line L625 (986.9669, 229.5481) -> (986.8919, 229.6231)
  line L626 (986.8919, 229.6231) -> (986.8169, 229.6981)
  line L627 (986.8169, 229.6981) -> (986.7419, 229.7481)
  line L628 (986.7419, 229.7481) -> (986.642, 229.8231)
  line L629 (986.642, 229.8231) -> (986.567, 229.8732)
  line L630 (986.567, 229.8732) -> (986.467, 229.9232)
  line L631 (986.467, 229.9232) -> (986.367, 229.9733)
  line L632 (986.367, 229.9733) -> (986.267, 229.9983)
  line L633 (986.267, 229.9983) -> (986.1671, 230.0483)
  line L634 (986.1671, 230.0483) -> (986.0671, 230.0483)
  line L635 (986.0671, 230.0483) -> (985.9671, 230.0734)
  line L636 (985.9671, 230.0734) -> (985.8671, 230.0984)
  line L637 (985.8671, 230.0984) -> (985.7671, 230.0984)
  line L638 (985.7671, 230.0984) -> (985.6671, 230.0984)
  line L639 (985.6671, 230.0984) -> (985.5421, 230.0734)
  line L640 (985.5421, 230.0734) -> (985.4421, 230.0484)
  line L641 (985.4421, 230.0484) -> (985.3421, 230.0484)
  line L642 (985.3421, 230.0484) -> (985.2421, 229.9984)
  line L643 (985.2421, 229.9984) -> (985.1421, 229.9734)
  line L644 (985.1421, 229.9734) -> (985.0421, 229.9234)
  line L645 (985.0421, 229.9234) -> (984.9671, 229.8734)
  line L646 (984.9671, 229.8734) -> (984.8671, 229.8234)
  line L647 (984.8671, 229.8234) -> (984.7921, 229.7484)
  line L648 (984.7921, 229.7484) -> (984.7171, 229.6984)
  line L649 (984.7171, 229.6984) -> (984.6421, 229.6234)
  line L650 (984.6421, 229.6234) -> (984.5671, 229.5484)
  line L651 (984.5671, 229.5484) -> (984.492, 229.4734)
  line L652 (984.492, 229.4734) -> (984.4421, 229.3734)
  line L653 (984.4421, 229.3734) -> (984.3671, 229.2984)
  line L654 (984.3671, 229.2984) -> (984.317, 229.1985)
  line L655 (984.317, 229.1985) -> (984.292, 229.0984)
  line L656 (984.292, 229.0984) -> (984.2421, 228.9984)
  line L657 (984.2421, 228.9984) -> (984.2171, 228.8985)
  line L658 (984.2171, 228.8985) -> (984.192, 228.7984)
  line L659 (984.192, 228.7984) -> (984.167, 228.6984)
  line L660 (984.167, 228.6984) -> (984.167, 228.5984)
  line L661 (984.167, 228.5984) -> (984.167, 228.4984)
  line L662 (984.167, 228.4984) -> (984.167, 228.3984)
  line L663 (984.167, 228.3984) -> (984.167, 228.2734)
  line L664 (984.167, 228.2734) -> (984.192, 228.1735)
  line L665 (984.192, 228.1735) -> (984.2171, 228.0734)
  line L666 (984.2171, 228.0734) -> (984.2421, 227.9734)
  line L667 (984.2421, 227.9734) -> (984.292, 227.8735)
  line L668 (984.292, 227.8735) -> (984.317, 227.7734)
  line L669 (984.317, 227.7734) -> (984.3671, 227.6985)
  line L670 (984.3671, 227.6985) -> (984.4421, 227.5985)
  line L671 (984.4421, 227.5985) -> (984.4921, 227.5235)
  line L672 (984.4921, 227.5235) -> (984.5671, 227.4235)
  line L673 (984.5671, 227.4235) -> (984.6421, 227.3484)
  line L674 (984.6421, 227.3484) -> (984.7171, 227.2984)
  line L675 (984.7171, 227.2984) -> (984.7921, 227.2234)
  line L676 (984.7921, 227.2234) -> (984.867, 227.1483)
  line L677 (984.867, 227.1483) -> (984.967, 227.0983)
  line L678 (984.967, 227.0983) -> (985.042, 227.0483)
  line L679 (985.042, 227.0483) -> (985.1419, 227.0233)
  line L680 (985.1419, 227.0233) -> (985.2419, 226.9732)
  line L681 (985.2419, 226.9732) -> (985.3419, 226.9482)
  line L682 (985.3419, 226.9482) -> (985.4419, 226.9231)
  line L683 (985.4419, 226.9231) -> (985.542, 226.8981)
  line L684 (985.542, 226.8981) -> (985.6669, 226.8981)
  line L685 (985.6669, 226.8981) -> (985.7669, 226.8981)
  line L686 (985.7669, 226.8981) -> (985.8669, 226.8981)
  line L687 (985.8669, 226.8981) -> (985.9669, 226.8981)
  line L688 (985.9669, 226.8981) -> (986.0669, 226.9231)
  line L689 (986.0669, 226.9231) -> (986.1669, 226.9481)
  line L690 (986.1669, 226.9481) -> (986.2669, 226.9731)
  line L691 (986.2669, 226.9731) -> (986.3669, 227.0231)
  line L692 (986.3669, 227.0231) -> (986.4669, 227.0481)
  line L693 (986.4669, 227.0481) -> (986.5669, 227.0981)
  line L694 (986.5669, 227.0981) -> (986.6419, 227.1481)
  line L695 (986.6419, 227.1481) -> (986.7419, 227.2231)
  line L696 (986.7419, 227.2231) -> (986.8169, 227.2981)
  line L697 (986.8169, 227.2981) -> (986.8919, 227.3481)
  line L698 (986.8919, 227.3481) -> (986.9668, 227.4231)
  line L699 (986.9668, 227.4231) -> (987.0419, 227.5231)
  line L700 (987.0419, 227.5231) -> (987.0919, 227.5981)
  line L701 (987.0919, 227.5981) -> (987.1419, 227.6981)
  line L702 (987.1419, 227.6981) -> (987.1919, 227.7731)
  line L703 (987.1919, 227.7731) -> (987.242, 227.8731)
  line L704 (987.242, 227.8731) -> (987.267, 227.9731)
  line L705 (987.267, 227.9731) -> (987.3169, 228.0731)
  line L706 (987.3169, 228.0731) -> (987.3419, 228.1731)
  line L707 (987.3419, 228.1731) -> (987.3419, 228.2731)
  line L708 (987.3419, 228.2731) -> (987.3669, 228.3981)
  line L709 (987.3669, 228.3981) -> (987.3669, 228.4981)
  line L710 (987.3669, 228.4981) -> (987.3669, 228.598)
  line L711 (987.3669, 228.598) -> (987.3418, 228.698)
  line L712 (968.868, 231.9734) -> (968.6179, 232.5734)
  line L713 (968.6179, 232.5734) -> (968.218, 233.0984)
  line L714 (968.218, 233.0984) -> (967.6929, 233.4984)
  line L715 (967.6929, 233.4984) -> (967.093, 233.7484)
  line L716 (967.093, 233.7484) -> (966.443, 233.8234)
  line L717 (966.443, 233.8234) -> (965.793, 233.7484)
  line L718 (965.793, 233.7484) -> (965.1679, 233.4984)
  line L719 (965.1679, 233.4984) -> (964.6429, 233.0984)
  line L720 (964.6429, 233.0984) -> (964.243, 232.5734)
  line L721 (964.243, 232.5734) -> (963.9929, 231.9734)
  line L722 (963.9929, 231.9734) -> (963.9179, 231.2984)
  line L723 (963.9179, 231.2984) -> (963.9929, 230.6484)
  line L724 (963.9929, 230.6484) -> (964.243, 230.0484)
  line L725 (964.243, 230.0484) -> (964.643, 229.5234)
  line L726 (964.643, 229.5234) -> (965.1679, 229.1235)
  line L727 (965.1679, 229.1235) -> (965.793, 228.8735)
  line L728 (965.793, 228.8735) -> (966.443, 228.7986)
  line L729 (966.443, 228.7986) -> (967.093, 228.8736)
  line L730 (967.093, 228.8736) -> (967.6929, 229.1236)
  line L731 (967.6929, 229.1236) -> (968.218, 229.5236)
  line L732 (968.218, 229.5236) -> (968.618, 230.0486)
  line L733 (968.618, 230.0486) -> (968.868, 230.6486)
  line L734 (968.868, 230.6486) -> (968.9429, 231.2986)
  line L735 (968.9429, 231.2986) -> (968.868, 231.9734)
  line L736 (1021.9429, 238.0232) -> (1021.9178, 238.3482)
  line L737 (1021.9178, 238.3482) -> (1021.8678, 238.6732)
  line L738 (1021.8678, 238.6732) -> (1021.7928, 238.9732)
  line L739 (1021.7928, 238.9732) -> (1021.6927, 239.2982)
  line L740 (1021.6927, 239.2982) -> (1021.5928, 239.5982)
  line L741 (1021.5928, 239.5982) -> (1021.4429, 239.8983)
  line L742 (1021.4429, 239.8983) -> (1021.2928, 240.1983)
  line L743 (1021.2928, 240.1983) -> (1021.1178, 240.4732)
  line L744 (1021.1178, 240.4732) -> (1020.9178, 240.7232)
  line L745 (1020.9178, 240.7232) -> (1020.7178, 240.9982)
  line L746 (1020.7178, 240.9982) -> (1020.4929, 241.2233)
  line L747 (1020.4929, 241.2233) -> (1020.2679, 241.4483)
  line L748 (1020.2679, 241.4483) -> (1020.018, 241.6484)
  line L749 (1020.018, 241.6484) -> (1019.7431, 241.8485)
  line L750 (1019.7431, 241.8485) -> (1019.4681, 242.0235)
  line L751 (1019.4681, 242.0235) -> (1019.1682, 242.1737)
  line L752 (1019.1682, 242.1737) -> (1018.8681, 242.2987)
  line L753 (1018.8681, 242.2987) -> (1018.5682, 242.4237)
  line L754 (1018.5682, 242.4237) -> (1018.2682, 242.5238)
  line L755 (1018.2682, 242.5238) -> (1017.9432, 242.5989)
  line L756 (1017.9432, 242.5989) -> (1017.6182, 242.6489)
  line L757 (1017.6182, 242.6489) -> (1017.2933, 242.6739)
  line L758 (1017.2933, 242.6739) -> (1016.9682, 242.699)
  line L759 (1016.9682, 242.699) -> (949.7668, 242.699)
  line L760 (949.7668, 242.699) -> (949.7668, 182.6984)
  line L761 (949.7668, 182.6984) -> (1016.9668, 182.6984)
  line L762 (1016.9668, 182.6984) -> (1017.2919, 182.6984)
  line L763 (1017.2919, 182.6984) -> (1017.6168, 182.7234)
  line L764 (1017.6168, 182.7234) -> (1017.9418, 182.7984)
  line L765 (1017.9418, 182.7984) -> (1018.2668, 182.8734)
  line L766 (1018.2668, 182.8734) -> (1018.5668, 182.9484)
  line L767 (1018.5668, 182.9484) -> (1018.8668, 183.0734)
  line L768 (1018.8668, 183.0734) -> (1019.1668, 183.1985)
  line L769 (1019.1668, 183.1985) -> (1019.4668, 183.3485)
  line L770 (1019.4668, 183.3485) -> (1019.7418, 183.5235)
  line L771 (1019.7418, 183.5235) -> (1020.0167, 183.7236)
  line L772 (1020.0167, 183.7236) -> (1020.2666, 183.9237)
  line L773 (1020.2666, 183.9237) -> (1020.4917, 184.1486)
  line L774 (1020.4917, 184.1486) -> (1020.7167, 184.3986)
  line L775 (1020.7167, 184.3986) -> (1020.9168, 184.6485)
  line L776 (1020.9168, 184.6485) -> (1021.1168, 184.9235)
  line L777 (1021.1168, 184.9235) -> (1021.2919, 185.1985)
  line L778 (1021.2919, 185.1985) -> (1021.442, 185.4734)
  line L779 (1021.442, 185.4734) -> (1021.5921, 185.7733)
  line L780 (1021.5921, 185.7733) -> (1021.6922, 186.0733)
  line L781 (1021.6922, 186.0733) -> (1021.7924, 186.3983)
  line L782 (1021.7924, 186.3983) -> (1021.8674, 186.7233)
  line L783 (1021.8674, 186.7233) -> (1021.9176, 187.0482)
  line L784 (1021.9176, 187.0482) -> (1021.9427, 187.3732)
  line L785 (1021.9427, 187.3732) -> (1021.9678, 187.6982)
  line L786 (1021.9678, 187.6982) -> (1021.9678, 237.6982)
  line L787 (1021.9678, 237.6982) -> (1021.9429, 238.0232)
  point P0 (0, 0)
  constraints: 1576 end point, 413 parallel, 135 perpendicular, 7 collinear
extrude "Extrusion1" add sketch "Sketch1" along normal blind 6
sketch "Sketch2" plane through (0, 0, 0) normal (0, -1, 0) x (1, 0, 0)
  line L0 (-1016.9669, 226.8982) -> (-1016.542, 226.8982) projected
  line L1 (-1016.9669, 230.292) -> (-1016.9669, 226.8982)
  line L2 (-1016.542, 195.8982) -> (-1016.9669, 195.8982) projected
  line L3 (-1016.7545, 195.8982) -> (-1016.7545, 199.114)
  line L4 (-996.9803, 190.0525) -> (-996.9803, 186.9282)
  line L5 (-985.7745, 199.114) -> (-985.7545, 195.8981)
  line L6 (-985.9669, 195.8981) -> (-985.542, 195.8981) projected
  line L7 (-966.4429, 197.1985) -> (-967.0929, 197.0985) projected
  line L8 (-965.793, 192.2485) -> (-966.443, 192.1486) projected
  line L9 (-966.4429, 197.1985) -> (-966.443, 192.1486)
  line L10 (-966.443, 233.8234) -> (-967.093, 233.7484) projected
  line L11 (-966.443, 233.8234) -> (-966.443, 228.7986)
  line L12 (-985.5421, 230.0734) -> (-985.6671, 230.0984) projected
  line L13 (-985.6671, 230.0984) -> (-985.6671, 226.8981)
  line L14 (-985.9669, 226.8981) -> (-985.542, 226.8981) projected
  line L15 (-996.7422, 239.0984) -> (-997.1672, 239.0984) projected
  line L16 (-996.9547, 239.0984) -> (-996.9547, 235.9332)
  point P0 (0, 0)
  point P1 (-1016.9669, 228.5951)
  point P2 (-996.9547, 237.5158)
  point P3 (-985.6671, 228.4982)
  point P4 (-985.7645, 197.5061)
  point P5 (-996.9803, 188.4903)
  point P6 (-1016.7545, 197.5061)
  constraints: 16 end point, 9 midpoint, 5 vertical, 1 point on line
hole "Hole1" at (-1016.9669, 0, 228.5951) at (-996.9547, 0, 237.5158) at (-985.6671, 0, 228.4982) at (-985.7645, 0, 197.5061) at (-996.9803, 0, 188.4903) at (-1016.7545, 0, 197.5061) direction (0, 1, 0) diameter 3.2 end through all
sketch "Sketch3" plane through (0, 0, 0) normal (0, -1, 0) x (1, 0, 0)
  line L0 (-966.443, 192.1486) -> (-966.4429, 197.1985)
  line L1 (-966.4429, 197.1985) -> (-966.443, 228.7986)
  line L2 (-966.443, 228.7986) -> (-966.443, 233.8234)
  point P0 (0, 0)
  point P1 (-966.443, 231.311)
  point P2 (-966.4429, 194.6735)
  constraints: 6 end point, 2 midpoint
hole "Hole2" at (-966.443, 0, 231.311) at (-966.4429, 0, 194.6735) direction (0, 1, 0) diameter 5 end through all
sketch "Sketch4" plane through (0, 0, 0) normal (0, -1, 0) x (1, 0, 0)
  line L0 (-1012.7681, 212.9999) -> (-1012.7431, 213.7485) projected
  line L1 (-1012.7681, 212.9999) -> (-989.767, 212.9984)
  circle A0 centre (-1001.2675, 212.9992) radius 11.5094
  point P0 (0, 0)
  constraints: 2 end point, 1 centre point, 1 midpoint
extrude "Extrusion2" cut sketch "Sketch4" against normal blind 10
body "Solid1"
